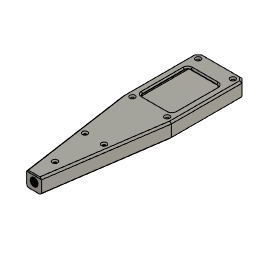
NFCTapHandle v7 (Autodesk Fusion 360 design; units mm, degrees)
Autodesk Fusion 360 part; units mm, degrees
sketch "Sketch1" plane through (0, 0, 0) normal (0, 0, 1) x (1, 0, 0)
  line L0 (0, 0) -> (47.55, 0) construction
  line L1 (47.55, 0) -> (47.55, 84.6) construction
  line L2 (47.55, 84.6) -> (0, 84.6) construction
  line L3 (0, 84.6) -> (0, 0) construction
  line L4 (3, 3) -> (44.55, 3) construction
  line L5 (44.55, 3) -> (44.55, 81.6) construction
  line L6 (44.55, 81.6) -> (3, 81.6) construction
  line L7 (3, 81.6) -> (3, 3) construction
  circle A0 centre (3, 81.6) radius 1.5
  circle A1 centre (44.55, 81.6) radius 1.5
  circle A2 centre (3, 3) radius 1.5
  circle A3 centre (44.55, 3) radius 1.5
  line L8 (4.275, 67.85) -> (43.275, 67.85)
  line L9 (43.275, 67.85) -> (43.275, 9.85)
  line L10 (43.275, 9.85) -> (4.275, 9.85)
  line L11 (4.275, 9.85) -> (4.275, 67.85)
  line L12 (23.775, 84.6) -> (23.775, 0) construction
  line L13 (23.775, 67.85) -> (23.775, 9.85) construction
  line L14 (-5, 84.6) -> (52.55, 84.6) construction
  line L15 (23.775, 84.6) -> (23.775, -135.4) construction
  line L16 (52.55, 84.6) -> (52.55, 0)
  line L17 (52.55, 0) -> (32.775, -135.4)
  line L18 (32.775, -135.4) -> (14.775, -135.4)
  line L19 (14.775, -135.4) -> (-5, 0)
  line L20 (-5, 0) -> (-5, 84.6)
  line L21 (-5, 84.6) -> (0, 89.6)
  line L22 (0, 89.6) -> (47.55, 89.6)
  line L23 (47.55, 89.6) -> (52.55, 84.6)
  line L24 (-0.2, -0.2) -> (47.75, -0.2)
  line L25 (47.75, -0.2) -> (47.75, 84.8)
  line L26 (47.75, 84.8) -> (-0.2, 84.8)
  line L27 (-0.2, 84.8) -> (-0.2, -0.2)
  line L28 (-0.2, 5.5) -> (47.75, 5.5)
  line L29 (-0.2, 79.1) -> (47.75, 79.1)
  line L30 (44.634, 1.1561) -> (25.8585, -127.4) construction
  line L31 (25.8585, -127.4) -> (21.6915, -127.4) construction
  line L32 (21.6915, -127.4) -> (2.916, 1.1561) construction
  circle A4 centre (12.3038, -63.1219) radius 1.5
  circle A5 centre (35.2462, -63.1219) radius 1.5
  circle A6 centre (23.775, -110.4) radius 1.5
  circle A7 centre (3, 81.6) radius 1.6
  circle A8 centre (44.55, 81.6) radius 1.6
  circle A9 centre (3, 3) radius 1.6
  circle A10 centre (23.775, -110.4) radius 1.6
  circle A11 centre (12.3038, -63.1219) radius 1.6
  circle A12 centre (35.2462, -63.1219) radius 1.6
  circle A13 centre (44.55, 3) radius 1.6
  dimension "d1" = 47.55
  dimension "d2" = 84.6
  dimension "d3" = -3
  dimension "d4" = 3
  dimension "d5" = 3
  dimension "d6" = 3
  dimension "d7" = 3
  dimension "d8" = 39
  dimension "d9" = 58
  dimension "d11" = 220
  dimension "d14" = 5
  dimension "d16" = 18
  dimension "d17" = 5
  dimension "d19" = 45
  dimension "d20" = 0.2
  dimension "d22" = 5.5
  dimension "d23" = 5.5
  dimension "d24" = 8
  dimension "d25" = 3
  dimension "d26" = 3
  dimension "d27" = 3
  dimension "d28" = 25
  dimension "d29" = 3.2
  dimension "d30" = 3.2
  dimension "d31" = 3.2
  dimension "d32" = 3.2
  dimension "d33" = 3.2
  dimension "d34" = 3.2
  dimension "d35" = 3.2
  dimension "d59" = 10.05
  constraint horizontal L0
  constraint vertical L1
  constraint horizontal L2
  constraint vertical L3
  constraint coincident L0.start L3.end
  constraint coincident L6.end L7.start
  constraint coincident L5.end L6.start
  constraint coincident L4.start L7.end
  constraint coincident L4.end L5.start
  constraint horizontal L8
  constraint vertical L9
  constraint horizontal L10
  constraint vertical L11
  constraint midpoint L2 L12.start
  constraint midpoint L0 L12.end
  constraint midpoint L8 L13.start
  constraint midpoint L10 L13.end
  constraint collinear L12 L13
  constraint parallel L2 L14
  constraint midpoint L14 L12.start
  constraint perpendicular L10 L15
  constraint collinear L12 L15
  constraint perpendicular L14 L16
  constraint perpendicular L14 L20
  constraint equal L17 L19
  constraint midpoint L15.end L18
  constraint perpendicular L15 L18
  constraint perpendicular L20 L22
  constraint equal L21 L23
  constraint horizontal L0.end L16.end
  constraint collinear L2 L14
  constraint coincident L27 L28.start
  constraint coincident L25 L28.end
  constraint perpendicular L25 L28
  constraint coincident L27 L29.start
  constraint perpendicular L16 L29
  constraint midpoint L32 A4.centre
  constraint midpoint L30 A5.centre
  constraint coincident L15 A6.centre
  constraint concentric A0 A7
  constraint concentric A1 A8
  constraint concentric A2 A9
  constraint concentric A6 A10
  constraint concentric A4 A11
  constraint concentric A5 A12
  constraint concentric A3 A13
  measures "d1" distance of L0.start L0.end
  measures "d2" distance of L0.start L2.end
  measures "d4" diameter of A0
  measures "d5" diameter of A1
  measures "d6" diameter of A2
  measures "d7" diameter of A3
  measures "d8" distance of L8.start L8.end
  measures "d9" distance of L8.start L10.end
  measures "d11" distance of L12.start L15.end
  measures "d14" distance of L1 L16
  measures "d16" distance of L17.end L18.end
  measures "d17" distance of L14 L22
  measures "d19" angle of L14 L23
  measures "d22" distance of L0 L28
  measures "d23" distance of L14 L29
  measures "d25" diameter of A4
  measures "d26" diameter of A5
  measures "d27" diameter of A6
  measures "d28" distance of L18 A6.centre
  measures "d29" diameter of A7
  measures "d30" diameter of A8
  measures "d31" diameter of A9
  measures "d32" diameter of A10
  measures "d33" diameter of A11
  measures "d34" diameter of A12
  measures "d35" diameter of A13
  measures "d59" distance of L10 L24
extrude "Extrude1" add sketch "Sketch1" along normal blind 2 contours L16 L17 L18 L19 L20 L21 L22 L23 | L24 L25 L27 L28 | L25 L27 L28 L29 | L25 L26 L27 L29 makes body 1
chamfer "Chamfer1" distance 1.5 angle 45 7 edges at (1.5083, 82.1786, 2) (1.5083, 3.5786, 2) (10.812, -62.5434, 2) (33.7545, -62.5434, 2) (22.2833, -109.8214, 2) (43.0583, 3.5786, 2) (43.0583, 82.1786, 2) on bodies 1
fillet "Fillet1" radius 4 4 edges at (4.275, 67.85, 1) (4.275, 9.85, 1) (43.275, 9.85, 1) (43.275, 67.85, 1) on bodies 1
chamfer "Chamfer2" distance 1.5 angle 45 8 edges at (4.275, 38.85, 2) (5.4466, 66.6784, 2) (23.775, 67.85, 2) (42.1034, 66.6784, 2) (43.275, 38.85, 2) (42.1034, 11.0216, 2) (23.775, 9.85, 2) (5.4466, 11.0216, 2) on bodies 1
extrude "Extrude6" add sketch "Sketch1" against normal blind 1.2 contours L24 L25 L27 L28 | L25 L26 L27 L29 bodies 1
chamfer "Chamfer5" distance 0.5 angle 45 8 edges at (47.75, 2.65, -1.2) (23.775, -0.2, -1.2) (23.775, 5.5, -1.2) (-0.2, 2.65, -1.2) (23.775, 79.1, -1.2) (47.75, 81.95, -1.2) (23.775, 84.8, -1.2) (-0.2, 81.95, -1.2) on bodies 1
extrude "Extrude2" add sketch "Sketch1" against normal blind 6 separate body contours L16 L17 L18 L19 L20 L21 L22 L23 makes body 2
extrude "Extrude3" add sketch "Sketch1" against normal blind 3.2 from surface at -2.8 contours L24 L25 L27 L28 | L25 L26 L27 L29 | A7 | A8 | A9 | A13 bodies 2
extrude "Extrude4" add sketch "Sketch1" against normal blind 10 from surface at -6 contours A0 | A1 | A2 | A3 | L8 L9 L10 L11 | L16 L17 L18 L19 L20 L21 L22 L23 | L24 L25 L27 L28 | L25 L27 L28 L29 | L25 L26 L27 L29 | A4 | A5 | A6 | A7 | A8 | A9 | A10 | A11 | A12 | A13 bodies 2
sketch "Sketch2" plane through (0, -135.4, 0) normal (0, -1, 0) x (1, 0, 0)
  line L0 (32.775, 0) -> (14.775, 0)
  line L1 (14.775, 0) -> (14.775, -16)
  line L2 (14.775, -16) -> (32.775, -16)
  line L3 (32.775, -16) -> (32.775, 0)
  line L4 (14.775, 0) -> (14.775, -16)
  line L5 (14.775, 0) -> (14.775, 2)
  line L6 (14.775, 2) -> (32.775, 2)
  line L7 (32.775, 0) -> (32.775, 2)
  line L8 (32.775, 0) -> (32.775, -16)
  line L9 (32.775, -16) -> (14.775, -16)
  line L10 (23.775, 2) -> (23.775, -16) construction
  circle A0 centre (23.775, -7) radius 4.7625
  dimension "d51" = 9.525
  constraint midpoint L6 L10.start
  constraint midpoint L9 L10.end
  constraint midpoint L10 A0.centre
  measures "d51" diameter of A0
chamfer "Chamfer3" distance 2 angle 45 7 edges at (42.6625, -67.7, -16) (52.55, 42.3, -16) (4.8875, -67.7, -16) (-5, 42.3, -16) (-2.5, 87.1, -16) (23.775, 89.6, -16) (50.05, 87.1, -16) on bodies 2
chamfer "Chamfer4" distance 2 angle 45 7 edges at (4.8875, -67.7, 2) (-5, 42.3, 2) (42.6625, -67.7, 2) (52.55, 42.3, 2) (-2.5, 87.1, 2) (23.775, 89.6, 2) (50.05, 87.1, 2) on bodies 1
thread "Thread1" "ISO Metric profile 3.0 M3x0.5 6H" major diameter 3.086 minor diameter 2.529 pitch 0.5 angle 60 modelled right hand crest width 0.1368 on face at (1.5905, 82.113, -4.9333) crest through (4.2645, 81.6, -2.925) on bodies 2
thread "Thread2" "ISO Metric profile 3.0 M3x0.5 6H" major diameter 3.086 minor diameter 2.529 pitch 0.5 angle 60 modelled right hand crest width 0.1368 on face at (46.0036, 81.9701, -4.9333) crest through (45.8145, 81.6, -2.925) on bodies 2
thread "Thread3" "ISO Metric profile 3.0 M3x0.5 6H" major diameter 3.086 minor diameter 2.529 pitch 0.5 angle 60 modelled right hand crest width 0.1368 on face at (4.4925, 2.8506, -3.8667) crest through (4.2645, 3, -2.925) on bodies 2
thread "Thread4" "ISO Metric profile 3.0 M3x0.5 6H" major diameter 3.086 minor diameter 2.529 pitch 0.5 angle 60 modelled right hand crest width 0.1368 on face at (46.0425, 2.8506, -3.8667) crest through (45.8145, 3, -2.925) on bodies 2
thread "Thread5" "ISO Metric profile 3.0 M3x0.5 6H" major diameter 3.086 minor diameter 2.529 pitch 0.5 angle 60 modelled right hand crest width 0.1368 on face at (11.2451, -64.3216, -4) crest through (13.5683, -63.1219, -0.125) on bodies 2
thread "Thread6" "ISO Metric profile 3.0 M3x0.5 6H" major diameter 3.086 minor diameter 2.529 pitch 0.5 angle 60 modelled right hand crest width 0.1368 on face at (34.1876, -64.3216, -4) crest through (36.5107, -63.1219, -0.125) on bodies 2
thread "Thread7" "ISO Metric profile 3.0 M3x0.5 6H" major diameter 3.086 minor diameter 2.529 pitch 0.5 angle 60 modelled right hand crest width 0.1368 on face at (22.3698, -111.1652, -4) crest through (25.0395, -110.4, -0.125) on bodies 2
extrude "Extrude5" cut sketch "Sketch2" against normal blind 20 contours A0 bodies 2
thread "Thread8" "ANSI Unified Screw Threads 0.375 3/8-24 UNF 3B" major diameter 9.525 minor diameter 8.4734 pitch 1.0583 angle 60 modelled right hand crest width 0.2916 on face at (28.5316, -122.0667, -7.2374) crest through (28.0117, -135.1354, -7) on bodies 2
named bodies: "Cover", "Body"
